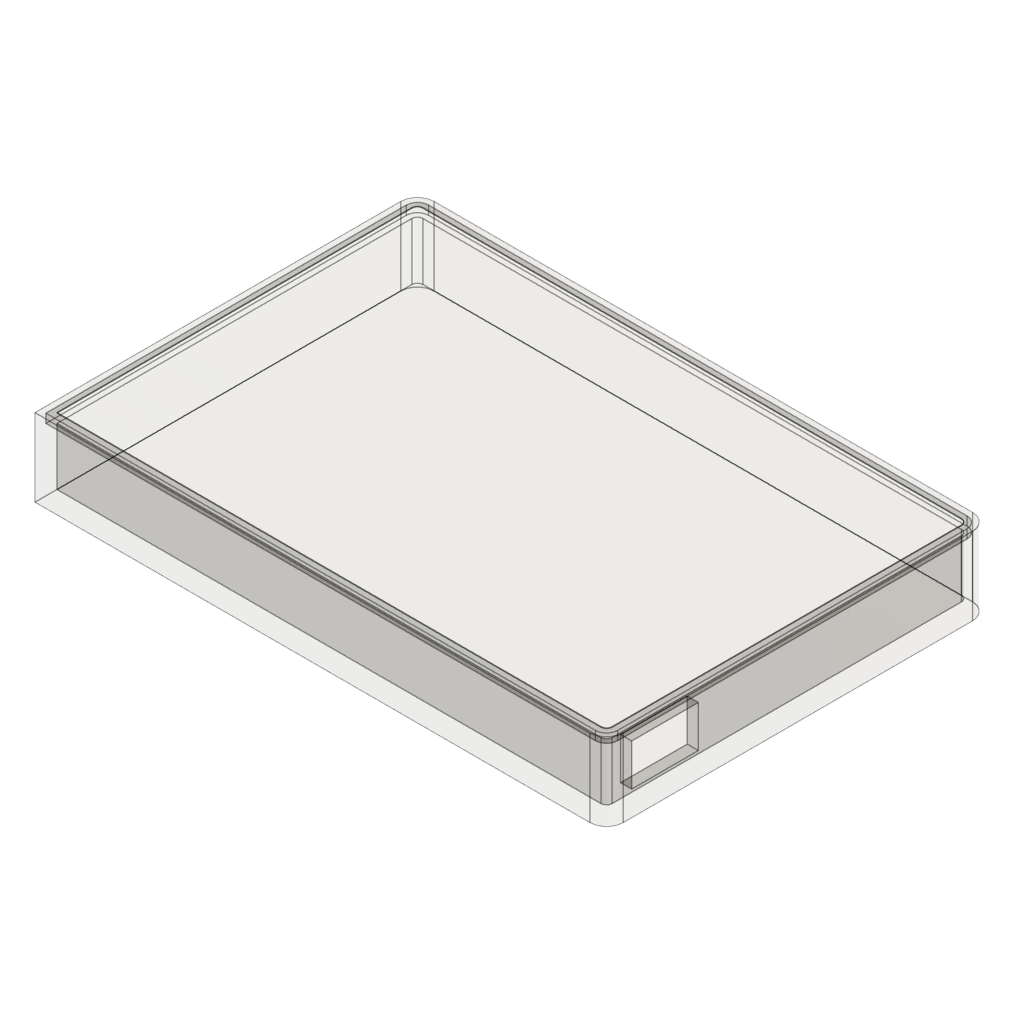
Caja_Collar (Autodesk Fusion 360 archive; units mm, degrees)
design "Caja_Base"
part number: 2026-10-04-12-38-26-154
Autodesk Fusion 360 part; units mm, degrees
other "DerivedContext1"
sketch "Boceto1" plane through (0, 0, 0) normal (0, 0, 1) x (1, 0, 0)
  line L0 (-0.0358, 2.4) -> (96.9103, 2.4)
  line L1 (99.9103, -0.6) -> (99.9103, -63.4961)
  line L2 (96.9103, -66.4961) -> (-3.0358, -66.4961)
  line L3 (-3.0358, -66.4961) -> (-3.0358, -0.6)
  arc A0 (-0.0358, 2.4) -> (-3.0358, -0.6) centre (-0.0358, -0.6) ccw
  arc A1 (99.9103, -0.6) -> (96.9103, 2.4) centre (96.9103, -0.6) ccw
  arc A2 (96.9103, -66.4961) -> (99.9103, -63.4961) centre (96.9103, -63.4961) ccw
  dimension "d2" = 3
  constraint horizontal L0
  constraint vertical L1
  constraint horizontal L2
  constraint vertical L3
  constraint tangent L0 A0
  constraint tangent L3 A0
  constraint tangent L0 A1
  constraint tangent L1 A1
  constraint equal A0 A1
  constraint tangent L1 A2
  constraint tangent L2 A2
  constraint equal A0 A2
  measures "d2" radius of A0
extrude "Extruir1" add sketch "Boceto1" against normal blind 14
shell "Vaciado1" thickness 2 removed faces 1 at (31.2795, -43.5308, 0)
ref_plane "PlanoDeObra1" through (48.4372, -32.0481, -1.7) normal (0, 0, 1) x (1, 0, 0)
sketch "Boceto3" plane through (0, 0, -1.7) normal (0, 0, 1) x (1, 0, 0)
  line L0 (-1.0358, -64.4961) -> (96.9103, -64.4961)
  arc A0 (96.9103, -64.4961) -> (97.9103, -63.4961) centre (96.9103, -63.4961) ccw
  line L1 (97.9103, -63.4961) -> (97.9103, -0.6)
  arc A1 (97.9103, -0.6) -> (96.9103, 0.4) centre (96.9103, -0.6) ccw
  line L2 (96.9103, 0.4) -> (-0.0358, 0.4)
  arc A2 (-0.0358, 0.4) -> (-1.0358, -0.6) centre (-0.0358, -0.6) ccw
  line L3 (-1.0358, -0.6) -> (-1.0358, -64.4961)
  line L4 (-2.0358, -0.6) -> (-2.0358, -65.4961)
  line L5 (-2.0358, -65.4961) -> (96.9103, -65.4961)
  arc A3 (96.9103, -65.4961) -> (98.9103, -63.4961) centre (96.9103, -63.4961) ccw
  line L6 (98.9103, -63.4961) -> (98.9103, -0.6)
  arc A4 (98.9103, -0.6) -> (96.9103, 1.4) centre (96.9103, -0.6) ccw
  line L7 (96.9103, 1.4) -> (-0.0358, 1.4)
  arc A5 (-0.0358, 1.4) -> (-2.0358, -0.6) centre (-0.0358, -0.6) ccw
  dimension "d8" = 1
extrude "Extruir2" cut sketch "Boceto3" along normal blind 1.6 contours L0 A0 L1 A1 L2 A2 L3 | L4 L5 A3 L6 A4 L7 A5
sketch "sketch 1000" plane through (99.9103, 0, 0) normal (1, 0, 0) x (0, 1, 0)
  line L0 (-0.6, 0) -> (-63.4961, 0)
  line L1 (-63.4961, 0) -> (-63.4961, -14)
  line L2 (-63.4961, -14) -> (-0.6, -14)
  line L3 (-0.6, -14) -> (-0.6, 0)
  line L4 (-61.9707, -2) -> (-49.9707, -2)
  line L5 (-49.9707, -2) -> (-49.9707, -9.5)
  line L6 (-49.9707, -9.5) -> (-61.9707, -9.5)
  line L7 (-61.9707, -9.5) -> (-61.9707, -2)
extrude "Extruir3" cut sketch "sketch 1000" against normal blind 4 contours L4 L5 L6 L7
